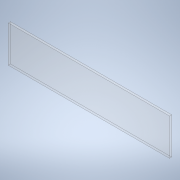
# Autodesk Inventor part: arm1
Saved by Autodesk Inventor 2021 (Build 250183000, 183)
## iProperties
Created: 2022-05-21
Part Number: arm1
Material: Polycarbonate, Clear
Document SubType Name: Modeling
Designer: techv
Mass: 44.8982 g
Surface Area: 268.565 cm^2
Volume: 37.4152 cm^3
Density: 1.2 g/cm^3
Appearance: Polycarbonate - Clear
Author: techv
Autodesk Inventor part; units mm, degrees
ref_plane "YZ Plane" through (0, 0, 0) normal (1, 0, 0) x (0, 1, 0)
ref_plane "XZ Plane" through (0, 0, 0) normal (0, 1, 0) x (-1, 0, 0)
ref_plane "XY Plane" through (0, 0, 0) normal (0, 0, 1) x (1, 0, 0)
sketch "Sketch1" plane through (0, 0, 0) normal (0, 0, 1) x (1, 0, 0)
  circle A0 centre (6.0619, 42.5) radius 1.5 projected
  circle A1 centre (6.0619, 7.5) radius 1.5 projected
  circle A2 centre (28.8092, 42.5) radius 1.5 projected
  circle A3 centre (28.8092, 7.5) radius 1.5 projected
  line L0 (34.8712, 0) -> (0, 0) projected
  line L1 (34.8712, 0) -> (34.8712, 50) projected
  line L2 (0, 50) -> (34.8712, 50) projected
  line L3 (0, 0) -> (0, 50) projected
  line L4 (0, 0) -> (220, 0)
  line L5 (220, 0) -> (220, 50)
  line L6 (220, 50) -> (0, 50)
  line L7 (0, 50) -> (0, 0)
  point P0 (19, 50)
  point P1 (19, 0)
  dimension "d0" = 220
  dimension "d1" = 50
  constraints: 8 end point, 2 parallel, 1 horizontal, 1 perpendicular
  measures "d0" distance of L6.end L5.end
  measures "d1" distance of L5.end L4.end
extrude "Extrusion1" add sketch "Sketch1" along normal blind 3 contours A0 | A1 | A2 | A3 | L0 L3 L2 L1 | L1 L6 L5 L4
body "Solid1"
